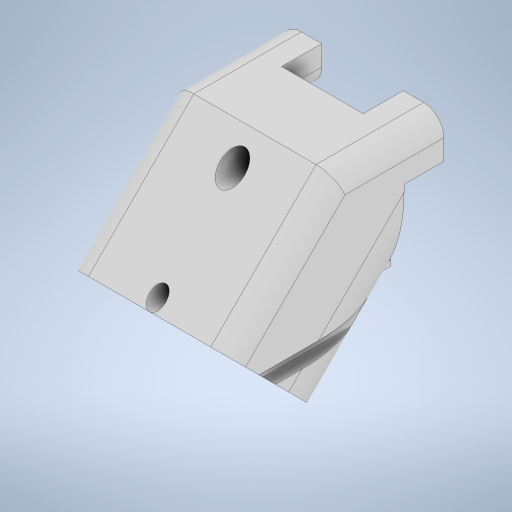
# Autodesk Inventor part: Fingertip End
Saved by Autodesk Inventor 2023 (Build 270158000, 158)
## iProperties
Created: 2023-04-06
Part Number: Fingertip End
Material: Generic
Document SubType Name: Modeling
Designer: 1roweste
Density: 1 g/cm^3
Appearance: Default
Author: 1roweste
Autodesk Inventor part; units mm, degrees
sketch "Connection Imprint" plane through (0, 0, 0) normal (0, 0, 1) x (1, 0, 0)
  line L0 (-1, 8.6927) -> (-1, -8.6927)
  arc A0 (1, 8.6927) -> (-1, 8.6927) centre (0, 0) ccw
  line L1 (1, -8.6927) -> (1, 8.6927)
  arc A1 (-1, -8.6927) -> (1, -8.6927) centre (0, 0) ccw
  line L2 (-5, 10) -> (-5, 7.5)
  arc A2 (-7.5, 5) -> (-5, 7.5) centre (-7.5, 7.5) ccw
  line L3 (-7.5, 5) -> (-10, 5)
  line L4 (-10, 0) -> (-10, 5)
  arc A3 (-10, 0) -> (-3.5, -9.3675) centre (0, 0) ccw
  line L5 (-3.5, -9.3675) -> (-3.5, -8.6927)
  line L6 (-3.5, -8.6927) -> (-2, -8.6927)
  line L7 (-2, -8.6927) -> (-2, -9.798)
  arc A4 (-2, -9.798) -> (2, -9.798) centre (0, 0) ccw
  line L8 (2, -9.798) -> (2, -8.6927)
  line L9 (2, -8.6927) -> (3.5, -8.6927)
  line L10 (3.5, -8.6927) -> (3.5, -9.3675)
  arc A5 (3.5, -9.3675) -> (10, 0) centre (0, 0) ccw
  line L11 (10, 5) -> (10, 0)
  line L12 (10, 5) -> (7.5, 5)
  arc A6 (5, 7.5) -> (7.5, 5) centre (7.5, 7.5) ccw
  line L13 (5, 7.5) -> (5, 10)
  line L14 (-5, 10) -> (5, 10)
  arc A7 (-7.5, 5) -> (-5, 7.5) centre (-7.5, 7.5) ccw
  line L15 (-5, 10) -> (-5, 7.5)
  line L16 (-7.5, 10) -> (-5, 10)
  arc A8 (-7.5, 10) -> (-10, 7.5) centre (-7.5, 7.5) ccw
  line L17 (-10, 5) -> (-10, 7.5)
  line L18 (-7.5, 5) -> (-10, 5)
  arc A9 (10, 7.5) -> (7.5, 10) centre (7.5, 7.5) ccw
  line L19 (5, 10) -> (7.5, 10)
  line L20 (5, 7.5) -> (5, 10)
  arc A10 (5, 7.5) -> (7.5, 5) centre (7.5, 7.5) ccw
  line L21 (10, 5) -> (7.5, 5)
  line L22 (10, 7.5) -> (10, 5)
  line L23 (2, -9.798) -> (2, -8.6927)
  arc A11 (2, -9.798) -> (3.5, -9.3675) centre (0, 0) ccw
  line L24 (3.5, -8.6927) -> (3.5, -9.3675)
  line L25 (2, -8.6927) -> (3.5, -8.6927)
  line L26 (-3.5, -9.3675) -> (-3.5, -8.6927)
  arc A12 (-3.5, -9.3675) -> (-2, -9.798) centre (0, 0) ccw
  line L27 (-2, -8.6927) -> (-2, -9.798)
  line L28 (-3.5, -8.6927) -> (-2, -8.6927)
  constraints: 58 end point, 26 point on circle, 13 centre point
extrude "Extrusion1" add sketch "Connection Imprint" along normal blind 4.9 contours L2 A2 L3 L17 A8 L16 | L19 A9 L22 L12 A6 L13 | L5 L6 L7 A12 | A11 L8 L9 L10
sketch "Plane Rotational Axis" plane through (0, 0, 0) normal (0, 0, -1) x (-1, 0, 0)
  arc A0 (-2, -9.798) -> (2, -9.798) centre (0, 0) ccw projected
  line L0 (-1, -8.6927) -> (-1, 8.6927) projected
  line L1 (0, -10) -> (-1, -10)
  constraints: 2 end point, 1 perpendicular, 1 point on circle, 1 point on line, 1 tangent
ref_plane "Rotational Plane" through (0, -10, 0) normal (0, 0.7071068, 0.7071068) x (1, 0, 0)
sketch "Sketch3" plane through (0, -10, 0) normal (0, 0.7071068, 0.7071068) x (1, 0, 0)
  line L0 (-5, 20) -> (-5, 17.5)
  arc A0 (-7.5, 15) -> (-5, 17.5) centre (-7.5, 17.5) ccw
  line L1 (-7.5, 15) -> (-10, 15)
  line L2 (-10, 10) -> (-10, 15)
  arc A1 (-10, 10) -> (-3.5, 0.6325) centre (0, 10) ccw
  arc A2 (-2, 0.202) -> (2, 0.202) centre (0, 10) ccw
  line L3 (2, 0.202) -> (2, 1.3073)
  line L4 (2, 1.3073) -> (3.5, 1.3073)
  line L5 (3.5, 1.3073) -> (3.5, 0.6325)
  arc A3 (3.5, 0.6325) -> (10, 10) centre (0, 10) ccw
  line L6 (10, 15) -> (10, 10)
  line L7 (10, 15) -> (7.5, 15)
  arc A4 (5, 17.5) -> (7.5, 15) centre (7.5, 17.5) ccw
  line L8 (5, 17.5) -> (5, 20)
  line L9 (-5, 20) -> (5, 20)
  arc A5 (-7.5, 15) -> (-5, 17.5) centre (-7.5, 17.5) ccw
  line L10 (-5, 20) -> (-5, 17.5)
  line L11 (-7.5, 20) -> (-5, 20)
  arc A6 (-7.5, 20) -> (-10, 17.5) centre (-7.5, 17.5) ccw
  line L12 (-10, 15) -> (-10, 17.5)
  line L13 (-7.5, 15) -> (-10, 15)
  arc A7 (10, 17.5) -> (7.5, 20) centre (7.5, 17.5) ccw
  line L14 (5, 20) -> (7.5, 20)
  line L15 (5, 17.5) -> (5, 20)
  arc A8 (5, 17.5) -> (7.5, 15) centre (7.5, 17.5) ccw
  line L16 (10, 15) -> (7.5, 15)
  line L17 (10, 17.5) -> (10, 15)
  line L18 (2, 0.202) -> (2, 1.3073)
  arc A9 (2, 0.202) -> (3.5, 0.6325) centre (0, 10) ccw
  line L19 (3.5, 1.3073) -> (3.5, 0.6325)
  line L20 (2, 1.3073) -> (3.5, 1.3073)
  arc A10 (-3.5, 0.6325) -> (-2, 0.202) centre (0, 10) ccw
  line L21 (0, 0) -> (1, 0) projected
  point P0 (0, 7.0711)
  point P1 (0, 0)
  point P2 (-3.5, 0.6325)
  point P3 (2, 0.202)
  point P4 (3.5, 0.6325)
  point P5 (10, 15)
  point P6 (5, 20)
  point P7 (-10, 15)
  dimension "d3" = 0
  dimension "d4" = 0
  dimension "d5" = 0
  dimension "d6" = 0
  dimension "d8" = 0
  dimension "d9" = 0
  dimension "d10" = 0
  constraints: 42 end point, 23 point on circle, 11 centre point
  measures "d3" distance from line of point (0, 0) L21
  measures "d4" distance of L6.start L16.start
  measures "d5" distance of L1.end L12.start
  measures "d6" distance of A2.start A10.end
  measures "d8" distance of A10.start A1.end
  measures "d9" distance of L3.start L18.start
  measures "d10" vertical distance of L1.end L6.start
ref_plane "Extrusion BackstopOnDovetails" through (-3.5, -8.6927, 0) normal (0, 0, -1) x (-1, 0, 0)
extrude "Extrusion2" add sketch "Sketch3" along normal up to surface surface through (-3.5, -8.6927, 0) normal (0, 0, -1)
sketch "Sketch4" plane through (-3.5, -8.6927, 0) normal (0, 0, -1) x (-1, 0, 0)
  line L0 (-13.5, 13.6927) -> (-13.5, 8.6927) projected
  line L1 (-13.5, 16.1927) -> (-13.5, 13.6927) projected
  arc A0 (-11, 18.6927) -> (-13.5, 16.1927) centre (-11, 16.1927) ccw projected
  line L2 (1.5, 18.6927) -> (-8.5, 18.6927) projected
  line L3 (4, 18.6927) -> (1.5, 18.6927) projected
  arc A1 (6.5, 16.1927) -> (4, 18.6927) centre (4, 16.1927) ccw projected
  line L4 (6.5, 13.6927) -> (6.5, 16.1927) projected
  line L5 (6.5, 8.6927) -> (6.5, 13.6927) projected
  arc A2 (0, -0.6748) -> (6.5, 8.6927) centre (-3.5, 8.6927) ccw projected
  arc A3 (-5.5, -1.1053) -> (-1.5, -1.1053) centre (-3.5, 8.6927) ccw projected
  arc A4 (-1.5, -1.1053) -> (0, -0.6748) centre (-3.5, 8.6927) ccw projected
  arc A5 (-13.5, 8.6927) -> (-7, -0.6748) centre (-3.5, 8.6927) ccw projected
  arc A6 (-7, -0.6748) -> (-5.5, -1.1053) centre (-3.5, 8.6927) ccw projected
  line L6 (-13.5, 16.1927) -> (6.5, 16.1927)
  line L7 (6.5, 16.1927) -> (6.5, 31.1927)
  line L8 (6.5, 31.1927) -> (-13.5, 31.1927)
  line L9 (-13.5, 31.1927) -> (-13.5, 16.1927)
  line L10 (-8.5, 18.6927) -> (-8.5, 16.1927) projected
  line L11 (-11, 18.6927) -> (-8.5, 18.6927) projected
  line L12 (1.5, 16.1927) -> (1.5, 18.6927) projected
  dimension "d13" = 20
  dimension "d14" = 15
  constraints: 8 end point, 2 parallel, 1 horizontal, 1 perpendicular
  measures "d13" distance of L8.end L7.end
  measures "d14" distance of L7.end L6.end
extrude "Extrusion3" cut sketch "Sketch4" along normal blind 15 contours L9 L8 L7 A1 L3 L2 L11 A0
sketch "Sketch5" plane through (0, -10, 0) normal (0, -0.7071068, -0.7071068) x (-1, 0, 0)
  arc A0 (0, 0) -> (10, 10) centre (0, 10) ccw projected
  line L0 (10, 17.5) -> (10, 10) projected
  arc A1 (10, 17.5) -> (7.5, 20) centre (7.5, 17.5) ccw projected
  line L1 (-7.5, 20) -> (7.5, 20) projected
  arc A2 (-7.5, 20) -> (-10, 17.5) centre (-7.5, 17.5) ccw projected
  line L2 (-10, 10) -> (-10, 17.5) projected
  arc A3 (-10, 10) -> (0, 0) centre (0, 10) ccw projected
  point P0 (0, 7.0711)
extrude "Extrusion4" add sketch "Sketch5" along normal blind 10
sketch "Sketch6" plane through (-10, 5, 0) normal (0, 0, 1) x (1, 0, 0)
  line L0 (9, 3.6927) -> (9, -13.6927) projected
  line L1 (11, -13.6927) -> (11, 3.6927) projected
  arc A0 (9, -13.6927) -> (11, -13.6927) centre (10, -5) ccw projected
  arc A1 (11, 3.6927) -> (9, 3.6927) centre (10, -5) ccw projected
  line L2 (2.5, -7.9289) -> (17.5, -7.9289) projected
  circle A2 centre (10, -6.9289) radius 1
  circle A3 centre (10, 2.25) radius 1.5
  point P0 (10, 3.75)
  dimension "d29" = 3
  dimension "d30" = 1.5
  constraints: 3 tangent, 2 centre point, 1 point on circle
  measures "d29" diameter of A3
  measures "d30" distance of point (10, 3.75) A3.centre
extrude "Extrusion5" cut sketch "Sketch6" against normal up to surface contours A3 L1 L0 | L0 A3 | A3 L1 | A2 surface through (7.5, 4.1421, -14.1421) normal (0, 0.7071068, -0.7071068)
sketch "Sketch7" plane through (10, 5, 4.9) normal (1, 0, 0) x (0, 0, -1)
  line L0 (24.3454, -9.6967) -> (19.0421, -15) projected
  line L1 (21.6938, -12.3483) -> (4.9, -12.3483)
  line L2 (4.9, -0.8579) -> (4.9, -14.1055) projected
  line L3 (21.6938, -11.3483) -> (4.9, -11.3483)
  line L4 (20.6938, -13.3483) -> (4.9, -13.3483)
  line L5 (21.6938, -11.3483) -> (22.6938, -11.3483)
  point P0 (4.9, -5)
  point P1 (4.9, -13.3483)
  point P2 (4.9, -11.3483)
  dimension "d23" = 1
  dimension "d24" = 1
  constraints: 8 end point, 3 point on line, 2 horizontal, 2 parallel, 1 midpoint
  measures "d23" distance between parallel lines of L1 L3
  measures "d24" distance between parallel lines of L1 L4
sketch "TipImprint (DNE)" plane through (0, -17.0711, -7.0711) normal (0, -0.7071068, -0.7071068) x (-1, 0, 0)
  arc A0 (-10, 10) -> (10, 10) centre (0, 10) ccw projected
  line L0 (10, 10) -> (10, 17.5) projected
  arc A1 (10, 17.5) -> (7.5, 20) centre (7.5, 17.5) ccw projected
  line L1 (7.5, 20) -> (-7.5, 20) projected
  arc A2 (-7.5, 20) -> (-10, 17.5) centre (-7.5, 17.5) ccw projected
  line L2 (-10, 17.5) -> (-10, 10) projected
  point P0 (0, 7.0711)
extrude "Extrusion7" cut sketch "Sketch7" against normal blind 1.5
ref_plane "Work Plane3" through (0, 5, 4.9) normal (1, 0, 0) x (0, 0, -1)
mirror "Mirror1" about plane through (0, 5, 4.9) normal (1, 0, 0) of "Extrusion7"
body "Solid1"
